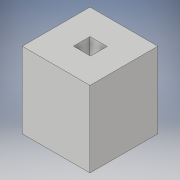
# Autodesk Inventor part: HeaderBlock
Saved by Autodesk Inventor 2019 (Build 230136000, 136)
## iProperties
Created: 2019-07-16
Part Number: HeaderBlock
Material: Generic
Document SubType Name: Modeling
Designer: james
Density: 1 g/cm^3
Appearance: Default
Author: james
Autodesk Inventor part; units mm, degrees
ref_plane "YZ Plane" through (0, 0, 0) normal (1, 0, 0) x (0, 1, 0)
ref_plane "XZ Plane" through (0, 0, 0) normal (0, 1, 0) x (-1, 0, 0)
ref_plane "XY Plane" through (0, 0, 0) normal (0, 0, 1) x (1, 0, 0)
sketch "Sketch1" plane through (0, 0, 0) normal (1, 0, 0) x (0, 1, 0)
  line L0 (1.463, 5.1734) -> (-1.377, 5.1734)
  line L1 (-1.377, 5.1734) -> (-1.377, 2.6334)
  line L2 (-1.377, 2.6334) -> (1.463, 2.6334)
  line L3 (1.463, 2.6334) -> (1.463, 5.1734)
  point P0 (0, 0)
  dimension "d0" = 2.54
  dimension "d1" = 2.84
  constraints: 8 end point, 2 parallel, 1 horizontal, 1 perpendicular
  measures "d0" distance of L2.end L0.start
  measures "d1" distance of L0.start L0.end
extrude "Extrusion1" add sketch "Sketch1" along normal blind 2.54
sketch "Sketch2" plane through (0, 1.463, 5.1734) normal (0, 1, 0) x (1, 0, 0)
  line L0 (0.96, 0.96) -> (1.6, 0.96)
  line L1 (1.6, 0.96) -> (1.6, 1.58)
  line L2 (1.6, 1.58) -> (0.96, 1.58)
  line L3 (0.96, 1.58) -> (0.96, 0.96)
  line L4 (0, 0) -> (2.54, 0) projected
  line L5 (0, 2.54) -> (2.54, 2.54) projected
  line L6 (0, 2.54) -> (0, 0) projected
  line L7 (2.54, 2.54) -> (2.54, 0) projected
  line L8 (2.54, 0) -> (2.54, 2.54) projected
  point P0 (0, 5.1734)
  dimension "d4" = 0.62
  dimension "d5" = 0.64
  dimension "d6" = 0.96
  dimension "d7" = 0.96
  dimension "d8" = 0.96
  dimension "d9" = 0.94
  constraints: 8 end point, 2 parallel, 1 horizontal, 1 perpendicular
  measures "d4" distance of L0.end L1.end
  measures "d5" distance of L1.end L2.end
  measures "d6" distance between parallel lines of L4 L0
  measures "d7" distance between parallel lines of L5 L2
  measures "d8" distance between parallel lines of L6 L3
  measures "d9" distance between parallel lines of L7 L1
extrude "Extrusion2" cut sketch "Sketch2" against normal blind 3.81 contours L3 L2 L1 L0
body "Solid1"
